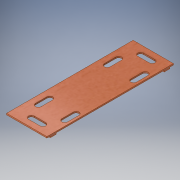
# Autodesk Inventor part: bett_V3_teil2_deckplatte_real
Saved by Autodesk Inventor 2018 (Build 220112000, 112)
## iProperties
Created: 2020-03-29
Part Number: bett_V3_teil2_deckplatte_real
Material: Holz (Walnuss)
Document SubType Name: Modeling
Designer: wepet
Density: 0.55 g/cm^3
Appearance: Walnuss - natur - poliert
Author: wepet
Autodesk Inventor part; units mm, degrees
ref_plane "YZ Plane" through (0, 0, 0) normal (1, 0, 0) x (0, 1, 0)
ref_plane "XZ Plane" through (0, 0, 0) normal (0, 1, 0) x (-1, 0, 0)
ref_plane "XY Plane" through (0, 0, 0) normal (0, 0, 1) x (1, 0, 0)
sketch "Skizze1" plane through (0, 0, 0) normal (0, 0, 1) x (1, 0, 0)
  line L0 (0, 0) -> (35, 0)
  line L1 (35, 0) -> (35, 110)
  line L2 (35, 110) -> (0, 110)
  line L3 (0, 110) -> (0, 0)
  line L4 (14, 105) -> (24, 105)
  line L5 (24, 105) -> (24, 100) construction
  line L6 (24, 100) -> (14, 100)
  line L7 (14, 100) -> (14, 105) construction
  line L8 (14, 10) -> (24, 10)
  line L9 (24, 10) -> (24, 5) construction
  line L10 (24, 5) -> (14, 5)
  line L11 (14, 5) -> (14, 10) construction
  line L12 (5, 90) -> (10, 90) construction
  line L13 (10, 90) -> (10, 80)
  line L14 (10, 80) -> (5, 80) construction
  line L15 (5, 80) -> (5, 90)
  line L16 (5, 30) -> (10, 30) construction
  line L17 (10, 30) -> (10, 20)
  line L18 (10, 20) -> (5, 20) construction
  line L19 (5, 20) -> (5, 30)
  line L20 (28, 90) -> (33, 90) construction
  line L21 (33, 90) -> (33, 80)
  line L22 (33, 80) -> (28, 80) construction
  line L23 (28, 80) -> (28, 90)
  line L24 (28, 30) -> (33, 30) construction
  line L25 (33, 30) -> (33, 20)
  line L26 (33, 20) -> (28, 20) construction
  line L27 (28, 20) -> (28, 30)
  line L28 (10, 80) -> (10, 30) construction
  line L29 (0, 55) -> (35, 55) construction
  arc A0 (5, 80) -> (10, 80) centre (7.5, 80) ccw
  arc A1 (10, 90) -> (5, 90) centre (7.5, 90) ccw
  arc A2 (33, 90) -> (28, 90) centre (30.5, 90) ccw
  arc A3 (28, 80) -> (33, 80) centre (30.5, 80) ccw
  arc A4 (24, 5) -> (24, 10) centre (24, 7.5) ccw
  arc A5 (14, 10) -> (14, 5) centre (14, 7.5) ccw
  arc A6 (5, 20) -> (10, 20) centre (7.5, 20) ccw
  arc A7 (28, 20) -> (33, 20) centre (30.5, 20) ccw
  arc A8 (33, 30) -> (28, 30) centre (30.5, 30) ccw
  arc A9 (10, 30) -> (5, 30) centre (7.5, 30) ccw
  arc A10 (24, 100) -> (24, 105) centre (24, 102.5) ccw
  arc A11 (14, 105) -> (14, 100) centre (14, 102.5) ccw
  line L30 (19, 10) -> (19, 100) construction
  line L31 (10, 85) -> (28, 85) construction
  point P0 (10, 55)
  point P1 (19, 85)
  dimension "d0" = 35
  dimension "d1" = 110
  dimension "d4" = 10
  dimension "d5" = 10
  dimension "d6" = 10
  dimension "d7" = 5
  dimension "d8" = 5
  dimension "d9" = 5
  dimension "d10" = 5
  dimension "d11" = 5
  dimension "d12" = 2
  dimension "d13" = 5
  dimension "d14" = 50
  dimension "d15" = 5
  constraints: 64 end point, 24 point on circle, 20 midpoint, 14 parallel, 12 centre point, 12 point on line, 7 horizontal, 7 perpendicular, 1 collinear, 1 tangent
  measures "d0" distance of L2.end L1.end
  measures "d1" distance of L1.end L0.end
  measures "d4" distance of L9.end L10.end
  measures "d5" distance of L18.end L16.start
  measures "d6" distance of L14.end L12.start
  measures "d7" distance of L17.end L18.end
  measures "d8" distance of L25.end L26.end
  measures "d9" distance of L8.end L9.end
  measures "d10" distance of L4.end L5.end
  measures "d11" distance between parallel lines of L2 L4
  measures "d12" distance between parallel lines of L1 L21
  measures "d13" distance between parallel lines of L3 L15
  measures "d14" distance between parallel lines of L14 L16
  measures "d15" distance between parallel lines of L0 L10
extrude "Extrusion2" add sketch "Skizze1" along normal blind 1.2
sketch "Skizze2" plane through (0, 0, 0) normal (0, 0, -1) x (-1, 0, 0)
  arc A0 (-28, 30) -> (-33, 30) centre (-30.5, 30) ccw construction
  line L0 (-28, 30) -> (-28, 20) construction
  arc A1 (-33, 20) -> (-28, 20) centre (-30.5, 20) ccw construction
  line L1 (-33, 20) -> (-33, 30) construction
  arc A2 (-28, 90) -> (-33, 90) centre (-30.5, 90) ccw construction
  line L2 (-28, 90) -> (-28, 80) construction
  arc A3 (-33, 80) -> (-28, 80) centre (-30.5, 80) ccw construction
  line L3 (-33, 80) -> (-33, 90) construction
  arc A4 (-5, 30) -> (-10, 30) centre (-7.5, 30) ccw construction
  line L4 (-5, 30) -> (-5, 20) construction
  arc A5 (-10, 20) -> (-5, 20) centre (-7.5, 20) ccw construction
  line L5 (-10, 20) -> (-10, 30) construction
  arc A6 (-5, 90) -> (-10, 90) centre (-7.5, 90) ccw construction
  line L6 (-5, 90) -> (-5, 80) construction
  arc A7 (-10, 80) -> (-5, 80) centre (-7.5, 80) ccw construction
  line L7 (-10, 80) -> (-10, 90) construction
  arc A8 (-24, 10) -> (-24, 5) centre (-24, 7.5) ccw construction
  line L8 (-24, 10) -> (-14, 10) construction
  arc A9 (-14, 5) -> (-14, 10) centre (-14, 7.5) ccw construction
  line L9 (-14, 5) -> (-24, 5) construction
  arc A10 (-24, 105) -> (-24, 100) centre (-24, 102.5) ccw construction
  line L10 (-24, 105) -> (-14, 105) construction
  arc A11 (-14, 100) -> (-14, 105) centre (-14, 102.5) ccw construction
  line L11 (-14, 100) -> (-24, 100) construction
  line L12 (0, 0) -> (-35, 0) construction
  line L13 (0, 110) -> (0, 0) construction
  line L14 (-35, 110) -> (0, 110) construction
  line L15 (-35, 0) -> (-35, 110) construction
  line L16 (-35, 3) -> (-30, 3)
  line L17 (-30, 3) -> (-30, 8)
  line L18 (-30, 8) -> (-35, 8)
  line L19 (-35, 8) -> (-35, 3)
  line L20 (-3, 3) -> (-8, 3)
  line L21 (-8, 3) -> (-8, 8)
  line L22 (-8, 8) -> (-3, 8)
  line L23 (-3, 8) -> (-3, 3)
  line L24 (-3, 102) -> (-8, 102)
  line L25 (-8, 102) -> (-8, 107)
  line L26 (-8, 107) -> (-3, 107)
  line L27 (-3, 107) -> (-3, 102)
  line L28 (-30, 107) -> (-35, 107)
  line L29 (-35, 107) -> (-35, 102)
  line L30 (-35, 102) -> (-30, 102)
  line L31 (-30, 102) -> (-30, 107)
  dimension "d18" = 5
  dimension "d19" = 5
  dimension "d20" = 5
  dimension "d21" = 5
  dimension "d22" = 3
  dimension "d23" = 0
  dimension "d24" = 3
  dimension "d25" = 3
  constraints: 32 end point, 8 parallel, 8 point on line, 4 horizontal, 4 perpendicular
  measures "d18" distance of L18.end L16.start
  measures "d19" distance of L16.start L16.end
  measures "d20" distance of L20.start L20.end
  measures "d21" distance of L28.end L29.end
  measures "d22" distance between parallel lines of L12 L16
  measures "d23" distance between parallel lines of L15 L19
  measures "d24" distance between parallel lines of L13 L23
  measures "d25" distance between parallel lines of L14 L28
extrude "Extrusion3" add sketch "Skizze2" along normal blind 1.2
